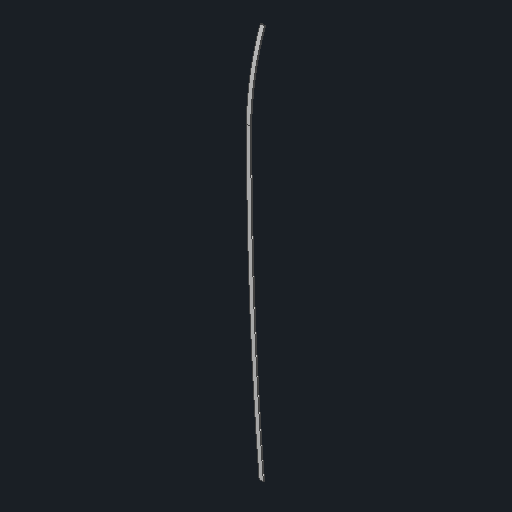
# Autodesk Inventor part: sealing_liner
Saved by Autodesk Inventor 2023 (Build 270158030, 158C)
## iProperties
Created: 2022-03-25
Part Number: sealing_liner
Material: Generic
Document SubType Name: Modeling
Designer: kardo
Density: 1 g/cm^3
Appearance: Default
Author: kardo
Autodesk Inventor part; units mm, degrees
ref_plane "YZ Plane" through (0, 0, 0) normal (1, 0, 0) x (0, 1, 0)
ref_plane "XZ Plane" through (0, 0, 0) normal (0, 1, 0) x (-1, 0, 0)
ref_plane "XY Plane" through (0, 0, 0) normal (0, 0, 1) x (1, 0, 0)
derived "parameters_frame.ipt"
derived "surface_body.ipt"
sketch "sk_rail_top_symmetry" plane through (0, 0, 0) normal (1, 0, 0) x (0, 1, 0)
  line L0 (0, 107.6209) -> (0, -224.5198) construction
  line L1 (0, 54.4) -> (-363, 54.4) construction
  line L2 (-363, 107.6209) -> (-363, -224.5198) construction
  line L3 (94.8, 107.6209) -> (94.8, -224.5198) construction
  line L4 (0, 54.4) -> (31.284, 54.4) construction
  line L5 (31.284, 54.4) -> (68.256, 47.9917) construction
  line L6 (68.256, 47.9917) -> (94.8, 37.536) construction
  line L7 (-487.5358, 0) -> (357.756, 0) construction
  spline S0 degree 2 poles (-363, 39.712) (-181.6483, 54.394) (0, 54.4) knots 0 0 0 1 1 1
  spline S1 degree 3 poles (0, 54.4) (31.284, 54.4) (68.256, 47.9917) (94.8, 37.536) knots 1 1 1 1 2 2 2 2
  point P0 (0, 0)
  point P1 (-181.5, 50.728)
  point P2 (94.8, 28.832)
ref_plane "plane_symmetry" through (0, 0, 0) normal (1, 0, 0) x (0, 1, 0)
sketch "sk_base" plane through (0, 0, 0) normal (1, 0, 0) x (0, 1, 0)
  spline S0 degree 2 poles (-363, 39.712) (-181.6483, 54.394) (0, 54.4) knots 0 0 0 1 1 1 projected
  spline S1 degree 3 poles (0, 54.4) (31.284, 54.4) (68.256, 47.9917) (94.8, 37.536) knots 1 1 1 1 2 2 2 2 projected
  line L0 (-362.9032, 38.5159) -> (-363, 39.712)
  line L1 (92.8, 38.3087) -> (92.3747, 37.1866)
  spline S2 degree 4 poles (-362.9032, 38.5159) (-272.3747, 45.845) (-181.6495, 50.7473) (-90.8247, 53.197) (0, 53.2) knots 0 0 0 0 0 1 1 1 1 1
  spline S3 degree 5 poles (0, 53.2) (9.8473, 53.1997) (19.6931, 52.6698) (29.5051, 51.7364) (48.1926, 49.2168) (66.6258, 45.2485) (75.3433, 43.0032) (83.9639, 40.374) (92.3747, 37.1865) knots 0 0 0 0 0 0 0.522625 0.522625 0.522625 1 1 1 1 1 1
  point P0 (0, 0)
  dimension "d7" = 1.2
  dimension "d8" = 2
  constraints: 4 end point, 9 other
  measures "d8" horizontal distance of point (94.8, 37.536) L1.start
extrude "thicken" add sketch "sk_base" along normal blind 5
equation "\"d7\" = cowl_liner_thickness"
equation "\"d8\" = bulkhead_thickness"
equation "\"d9\" = cowl_sealing_width"
equation "\"cowl_liner_thickness\" = 1.2"
equation "\"cowl_sealing_width\" = 5"
equation "\"bulkhead_thickness\" = 2"
body "Solid2"
